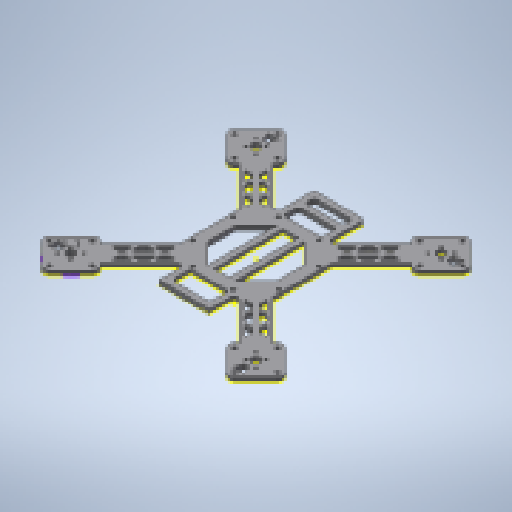
# Autodesk Inventor part: 顶板
Saved by Autodesk Inventor 2025.2 (Build 292293000, 293)
## iProperties
Created: 2025-10-21
Part Number: 顶板
Material: 常规
Document SubType Name: Modeling
Designer: BO‘S_SLAVE
Density: 1 g/cm^3
Appearance: 默认
Author: BO‘S_SLAVE
Autodesk Inventor part; units mm, degrees
ref_plane "YZ Plane" through (0, 0, 0) normal (1, 0, 0) x (0, 1, 0)
ref_plane "XZ Plane" through (0, 0, 0) normal (0, 1, 0) x (-1, 0, 0)
ref_plane "XY Plane" through (0, 0, 0) normal (0, 0, 1) x (1, 0, 0)
sketch "草图1" plane through (0, 0, 0) normal (0, 1, 0) x (-1, 0, 0)
  line L0 (27.5, 27.5) -> (-27.5, 27.5)
  line L1 (-27.5, 27.5) -> (-27.5, -27.5)
  line L2 (-27.5, -27.5) -> (27.5, -27.5)
  line L3 (27.5, -27.5) -> (27.5, 27.5)
  line L4 (77.7817, -77.7817) -> (-77.7817, 77.7817)
  line L5 (77.7817, 77.7817) -> (-77.7817, -77.7817)
  line L6 (0, 27.5) -> (0, -27.5)
  line L7 (27.5, 0) -> (-27.5, 0)
  line L8 (38.8909, 16.1091) -> (38.8909, -16.1091)
  line L9 (38.8909, -16.1091) -> (16.1091, -38.8909)
  line L10 (16.1091, -38.8909) -> (-16.1091, -38.8909)
  line L11 (-16.1091, -38.8909) -> (-38.8909, -16.1091)
  line L12 (-38.8909, -16.1091) -> (-38.8909, 16.1091)
  line L13 (-38.8909, 16.1091) -> (-16.1091, 38.8909)
  line L14 (-16.1091, 38.8909) -> (16.1091, 38.8909)
  line L15 (16.1091, 38.8909) -> (38.8909, 16.1091)
  line L16 (16.1091, -38.8909) -> (-16.1091, -38.8909)
  line L17 (-16.1091, 38.8909) -> (16.1091, 38.8909)
  line L18 (16.1091, 38.8909) -> (16.1091, 55)
  line L19 (-16.1091, 55) -> (-16.1091, 38.8909)
  line L20 (-70.7107, 84.8528) -> (-20.4289, 34.5711)
  line L21 (-34.5711, 20.4289) -> (-84.8528, 70.7107)
  line L22 (-84.8528, 70.7107) -> (-77.7817, 77.7817)
  line L23 (-77.7817, 77.7817) -> (-70.7107, 84.8528)
  line L24 (-53.033, 77.7817) -> (-77.7817, 53.033)
  line L25 (-77.7817, 53.033) -> (-102.5305, 77.7817)
  line L26 (-77.7817, 102.5305) -> (-53.033, 77.7817)
  line L27 (-53.033, 77.7817) -> (-102.5305, 77.7817) construction
  line L28 (-77.7817, 53.033) -> (-77.7817, 102.5305) construction
  line L29 (-11.3909, 27.5) -> (11.3909, 27.5)
  line L30 (11.3909, 27.5) -> (27.5, 11.3909)
  line L31 (27.5, 11.3909) -> (27.5, -11.3909)
  line L32 (27.5, -11.3909) -> (11.3909, -27.5)
  line L33 (11.3909, -27.5) -> (-11.3909, -27.5)
  line L34 (-11.3909, -27.5) -> (-27.5, -11.3909)
  line L35 (-27.5, -11.3909) -> (-27.5, 11.3909)
  line L36 (-27.5, 11.3909) -> (-11.3909, 27.5)
  line L37 (21.1091, 60) -> (21.1091, 33.8909)
  line L38 (-21.1091, 33.8909) -> (-21.1091, 60)
  circle A0 centre (-17, 36) radius 1.65
  line L39 (-38.8909, 0) -> (-27.5, 0)
  line L40 (0, 38.8909) -> (0, 27.5)
  line L41 (16.1091, 55) -> (-16.1091, 55)
  line L42 (21.1091, 60) -> (-21.1091, 60)
  circle A1 centre (-77.7817, 77.7817) radius 3.5
  circle A2 centre (-72.1249, 72.1249) radius 1.15
  circle A3 centre (-83.4386, 83.4386) radius 1.15
  circle A4 centre (-82.0244, 73.5391) radius 1.15
  circle A5 centre (-73.5391, 82.0244) radius 1.15
  circle A6 centre (-77.7817, 95.7817) radius 1.65
  circle A7 centre (-77.7817, 59.7817) radius 1.65
  circle A8 centre (-59.7817, 77.7817) radius 1.65
  circle A9 centre (-95.7817, 77.7817) radius 1.65
  line L43 (-77.7817, 102.5305) -> (-102.5305, 77.7817)
  line L44 (-77.7817, 102.5305) -> (-77.7817, 77.7817)
  line L45 (-77.7817, 77.7817) -> (-77.7817, 59.7817)
  line L46 (-73.5391, 82.0244) -> (-82.0244, 73.5391)
  line L47 (-72.1249, 72.1249) -> (-83.4386, 83.4386)
  line L48 (-20.4289, -34.5711) -> (-70.7107, -84.8528)
  line L49 (-84.8528, -70.7107) -> (-34.5711, -20.4289)
  line L50 (-77.7817, -53.033) -> (-53.033, -77.7817)
  line L51 (-102.5305, -77.7817) -> (-77.7817, -53.033)
  line L52 (-102.5305, -77.7817) -> (-77.7817, -102.5305)
  line L53 (-53.033, -77.7817) -> (-77.7817, -102.5305)
  line L54 (-82.0244, -73.5391) -> (-73.5391, -82.0244)
  circle A10 centre (-77.7817, -77.7817) radius 3.5
  circle A11 centre (-83.4386, -83.4386) radius 1.15
  circle A12 centre (-82.0244, -73.5391) radius 1.15
  circle A13 centre (-77.7817, -59.7817) radius 1.65
  circle A14 centre (-72.1249, -72.1249) radius 1.15
  circle A15 centre (-73.5391, -82.0244) radius 1.15
  circle A16 centre (-59.7817, -77.7817) radius 1.65
  circle A17 centre (-95.7817, -77.7817) radius 1.65
  circle A18 centre (-77.7817, -95.7817) radius 1.65
  line L55 (34.5711, -20.4289) -> (84.8528, -70.7107)
  line L56 (70.7107, -84.8528) -> (20.4289, -34.5711)
  line L57 (53.033, -77.7817) -> (77.7817, -53.033)
  line L58 (77.7817, -102.5305) -> (53.033, -77.7817)
  line L59 (77.7817, -102.5305) -> (102.5305, -77.7817)
  line L60 (77.7817, -53.033) -> (102.5305, -77.7817)
  line L61 (73.5391, -82.0244) -> (82.0244, -73.5391)
  circle A19 centre (77.7817, -77.7817) radius 3.5
  circle A20 centre (83.4386, -83.4386) radius 1.15
  circle A21 centre (73.5391, -82.0244) radius 1.15
  circle A22 centre (59.7817, -77.7817) radius 1.65
  circle A23 centre (72.1249, -72.1249) radius 1.15
  circle A24 centre (82.0244, -73.5391) radius 1.15
  circle A25 centre (77.7817, -59.7817) radius 1.65
  circle A26 centre (77.7817, -95.7817) radius 1.65
  circle A27 centre (95.7817, -77.7817) radius 1.65
  line L62 (20.4289, 34.5711) -> (70.7107, 84.8528)
  line L63 (84.8528, 70.7107) -> (34.5711, 20.4289)
  line L64 (77.7817, 53.033) -> (53.033, 77.7817)
  line L65 (102.5305, 77.7817) -> (77.7817, 53.033)
  line L66 (102.5305, 77.7817) -> (77.7817, 102.5305)
  line L67 (53.033, 77.7817) -> (77.7817, 102.5305)
  line L68 (82.0244, 73.5391) -> (73.5391, 82.0244)
  circle A28 centre (77.7817, 77.7817) radius 3.5
  circle A29 centre (83.4386, 83.4386) radius 1.15
  circle A30 centre (82.0244, 73.5391) radius 1.15
  circle A31 centre (77.7817, 59.7817) radius 1.65
  circle A32 centre (72.1249, 72.1249) radius 1.15
  circle A33 centre (73.5391, 82.0244) radius 1.15
  circle A34 centre (59.7817, 77.7817) radius 1.65
  circle A35 centre (95.7817, 77.7817) radius 1.65
  circle A36 centre (77.7817, 95.7817) radius 1.65
  circle A37 centre (-36, 17) radius 1.65
  circle A38 centre (-17, -36) radius 1.65
  circle A39 centre (-36, -17) radius 1.65
  circle A40 centre (17, 36) radius 1.65
  circle A41 centre (36, 17) radius 1.65
  circle A42 centre (36, -17) radius 1.65
  circle A43 centre (17, -36) radius 1.65
  line L69 (-19.4454, -19.4454) -> (-19.4454, 19.4454)
  line L70 (19.4454, -19.4454) -> (19.4454, 19.4454)
  line L71 (-16.1091, -38.8909) -> (-16.1091, -65)
  line L72 (-16.1091, -65) -> (16.1091, -65)
  line L73 (16.1091, -65) -> (16.1091, -38.8909)
  line L74 (-21.1091, -33.8909) -> (-21.1091, -70)
  line L75 (-21.1091, -70) -> (21.1091, -70)
  line L76 (21.1091, -70) -> (21.1091, -33.8909)
  line L77 (-16.1091, -56.9454) -> (16.1091, -56.9454)
  line L78 (-16.1091, -51.9454) -> (16.1091, -51.9454)
  line L79 (-11.5, 27.5) -> (-11.5, -27.5)
  line L80 (11.5, -27.5) -> (11.5, 27.5)
  line L81 (-6.5, -27.5) -> (-6.5, 27.5)
  line L82 (6.5, -27.5) -> (6.5, 27.5)
  line L83 (-63.9932, 66.8216) -> (-26.0858, 28.9142)
  line L84 (-66.8216, 63.9932) -> (-28.9142, 26.0858)
  line L85 (-58.3363, 72.4784) -> (-58.3363, 61.1647)
  line L86 (-56.3363, 70.4784) -> (-56.3363, 59.1647)
  line L87 (-42.1942, 56.3363) -> (-53.5079, 56.3363)
  line L88 (-40.1942, 54.3363) -> (-51.5079, 54.3363)
  line L89 (-40.1942, 54.3363) -> (-40.1942, 43.0226)
  line L90 (-38.1942, 52.2039) -> (-38.1942, 41.0226)
  line L91 (-35.3657, 38.1942) -> (-24.052, 38.1942)
  line L92 (-72.4784, 58.3363) -> (-61.1647, 58.3363)
  line L93 (-70.4784, 56.3363) -> (-59.1647, 56.3363)
  line L94 (-56.3363, 42.1942) -> (-56.3363, 53.5079)
  line L95 (-54.3363, 40.1942) -> (-54.3363, 51.5079)
  line L96 (-52.2039, 38.1942) -> (-41.0226, 38.1942)
  line L97 (-54.3363, 40.1942) -> (-43.0226, 40.1942)
  line L98 (-38.1942, 35.3657) -> (-38.1942, 24.052)
  line L99 (-70.3571, 60.4576) -> (-32.4497, 22.5503)
  line L100 (-60.4576, 70.3571) -> (-22.5503, 32.4497)
  line L101 (-38.1942, -35.3657) -> (-38.1942, -24.052)
  line L102 (-35.3657, -38.1942) -> (-24.052, -38.1942)
  line L103 (-38.1942, -52.2039) -> (-38.1942, -41.0226)
  line L104 (-40.1942, -54.3363) -> (-40.1942, -43.0226)
  line L105 (-52.2039, -38.1942) -> (-41.0226, -38.1942)
  line L106 (-54.3363, -40.1942) -> (-43.0226, -40.1942)
  line L107 (-60.4576, -70.3571) -> (-22.5503, -32.4497)
  line L108 (-42.1942, -56.3363) -> (-53.5079, -56.3363)
  line L109 (-40.1942, -54.3363) -> (-51.5079, -54.3363)
  line L110 (-56.3363, -70.4784) -> (-56.3363, -59.1647)
  line L111 (-58.3363, -72.4784) -> (-58.3363, -61.1647)
  line L112 (-63.9932, -66.8216) -> (-26.0858, -28.9142)
  line L113 (-66.8216, -63.9932) -> (-28.9142, -26.0858)
  line L114 (-70.4784, -56.3363) -> (-59.1647, -56.3363)
  line L115 (-72.4784, -58.3363) -> (-61.1647, -58.3363)
  line L116 (-70.3571, -60.4576) -> (-32.4497, -22.5503)
  line L117 (-56.3363, -42.1942) -> (-56.3363, -53.5079)
  line L118 (-54.3363, -40.1942) -> (-54.3363, -51.5079)
  line L119 (35.3657, -38.1942) -> (24.052, -38.1942)
  line L120 (38.1942, -35.3657) -> (38.1942, -24.052)
  line L121 (52.2039, -38.1942) -> (41.0226, -38.1942)
  line L122 (54.3363, -40.1942) -> (43.0226, -40.1942)
  line L123 (38.1942, -52.2039) -> (38.1942, -41.0226)
  line L124 (40.1942, -54.3363) -> (40.1942, -43.0226)
  line L125 (70.3571, -60.4576) -> (32.4497, -22.5503)
  line L126 (56.3363, -42.1942) -> (56.3363, -53.5079)
  line L127 (54.3363, -40.1942) -> (54.3363, -51.5079)
  line L128 (70.4784, -56.3363) -> (59.1647, -56.3363)
  line L129 (72.4784, -58.3363) -> (61.1647, -58.3363)
  line L130 (66.8216, -63.9932) -> (28.9142, -26.0858)
  line L131 (63.9932, -66.8216) -> (26.0858, -28.9142)
  line L132 (56.3363, -70.4784) -> (56.3363, -59.1647)
  line L133 (58.3363, -72.4784) -> (58.3363, -61.1647)
  line L134 (60.4576, -70.3571) -> (22.5503, -32.4497)
  line L135 (42.1942, -56.3363) -> (53.5079, -56.3363)
  line L136 (40.1942, -54.3363) -> (51.5079, -54.3363)
  line L137 (38.1942, 35.3657) -> (38.1942, 24.052)
  line L138 (35.3657, 38.1942) -> (24.052, 38.1942)
  line L139 (38.1942, 52.2039) -> (38.1942, 41.0226)
  line L140 (40.1942, 54.3363) -> (40.1942, 43.0226)
  line L141 (52.2039, 38.1942) -> (41.0226, 38.1942)
  line L142 (54.3363, 40.1942) -> (43.0226, 40.1942)
  line L143 (60.4576, 70.3571) -> (22.5503, 32.4497)
  line L144 (42.1942, 56.3363) -> (53.5079, 56.3363)
  line L145 (40.1942, 54.3363) -> (51.5079, 54.3363)
  line L146 (56.3363, 70.4784) -> (56.3363, 59.1647)
  line L147 (58.3363, 72.4784) -> (58.3363, 61.1647)
  line L148 (63.9932, 66.8216) -> (26.0858, 28.9142)
  line L149 (66.8216, 63.9932) -> (28.9142, 26.0858)
  line L150 (70.4784, 56.3363) -> (59.1647, 56.3363)
  line L151 (72.4784, 58.3363) -> (61.1647, 58.3363)
  line L152 (70.3571, 60.4576) -> (32.4497, 22.5503)
  line L153 (56.3363, 42.1942) -> (56.3363, 53.5079)
  line L154 (54.3363, 40.1942) -> (54.3363, 51.5079)
  line L155 (11.967, -28.8909) -> (-11.967, -28.8909)
  line L156 (-11.967, -28.8909) -> (-28.8909, -11.967)
  line L157 (-28.8909, -11.967) -> (-28.8909, 11.967)
  line L158 (-28.8909, 11.967) -> (-11.967, 28.8909)
  line L159 (-11.967, 28.8909) -> (11.967, 28.8909)
  line L160 (11.967, 28.8909) -> (28.8909, 11.967)
  line L161 (28.8909, 11.967) -> (28.8909, -11.967)
  line L162 (28.8909, -11.967) -> (11.967, -28.8909)
  line L163 (19.4454, -19.4454) -> (19.4454, -21.4124)
  line L164 (19.4454, 19.4454) -> (19.4454, 21.4124)
  line L165 (11.5, -27.5) -> (11.5, -28.8909)
  line L166 (6.5, -27.5) -> (6.5, -28.8909)
  line L167 (0, -27.5) -> (0, -28.8909)
  line L168 (19.4454, 19.4454) -> (19.4454, 21.4124)
  line L169 (11.5, 27.5) -> (11.5, 28.8909)
  line L170 (6.5, 27.5) -> (6.5, 28.8909)
  line L171 (0, 27.5) -> (0, 28.8909)
  line L172 (-19.4454, -19.4454) -> (-19.4454, -21.4124)
  line L173 (-19.4454, 19.4454) -> (-19.4454, 21.4124)
  line L174 (-11.5, -27.5) -> (-11.5, -28.8909)
  line L175 (-6.5, -27.5) -> (-6.5, -28.8909)
  line L176 (-11.5, 27.5) -> (-11.5, 28.8909)
  line L177 (-6.5, 27.5) -> (-6.5, 28.8909)
  line L178 (38.8909, -16.1091) -> (38.8909, -24.7487)
  line L179 (38.8909, 16.1091) -> (38.8909, 24.7487)
  line L180 (-38.8909, 16.1091) -> (-38.8909, 24.7487)
  line L181 (-38.8909, -24.7487) -> (-38.8909, -16.1091)
  line L182 (-83.7817, 77.7817) -> (-77.7817, 77.7817)
  line L183 (83.4484, 79.7817) -> (92.6247, 82.2405)
  line L184 (83.4484, 75.7817) -> (92.6247, 73.323)
  line L185 (83.4484, 75.7817) -> (83.4484, 79.7817)
  line L186 (77.7817, 77.7817) -> (77.7817, 102.5305)
  line L187 (84.9484, 75.3798) -> (84.9484, 80.1837)
  line L188 (83.4484, 77.7817) -> (77.7817, 77.7817)
  line L189 (92.6247, 73.323) -> (92.6247, 82.2405)
  line L190 (-75.7817, 83.4484) -> (-73.323, 92.6247)
  line L191 (-73.323, 92.6247) -> (-82.2405, 92.6247)
  line L192 (-79.7817, 83.4484) -> (-82.2405, 92.6247)
  line L193 (-75.3798, 84.9484) -> (-80.1837, 84.9484)
  line L194 (-75.7817, 83.4484) -> (-79.7817, 83.4484)
  line L195 (-83.4484, -75.7817) -> (-92.6247, -73.323)
  line L196 (-92.6247, -73.323) -> (-92.6247, -82.2405)
  line L197 (-83.4484, -79.7817) -> (-92.6247, -82.2405)
  line L198 (-84.9484, -75.3798) -> (-84.9484, -80.1837)
  line L199 (-83.4484, -75.7817) -> (-83.4484, -79.7817)
  line L200 (75.7817, -83.4484) -> (73.323, -92.6247)
  line L201 (73.323, -92.6247) -> (82.2405, -92.6247)
  line L202 (79.7817, -83.4484) -> (82.2405, -92.6247)
  line L203 (75.3798, -84.9484) -> (80.1837, -84.9484)
  line L204 (75.7817, -83.4484) -> (79.7817, -83.4484)
  arc A44 (88.4163, 74.97) -> (88.4163, 80.5935) centre (77.7817, 77.7817) ccw construction
  point P0 (0, 0)
  point P1 (0, 0)
  point P2 (0, 0)
  point P3 (0, 0)
  point P4 (-77.7817, 77.7817)
  point P5 (0, 0)
  point P6 (-72.4784, 58.3363)
  point P7 (22.5736, 37.4264)
  point P8 (-21.1091, 33.8909)
  point P9 (-59.7505, 71.0642)
  point P10 (16.1091, 38.8909)
  point P11 (-11.3909, 27.5)
  point P12 (11.3909, 27.5)
  point P13 (-77.7817, 77.7817)
  point P14 (-72.7259, 82.8376)
  point P15 (-74.0198, 81.0909)
  point P16 (-81.0909, 74.0198)
  point P17 (-82.8376, 72.7259)
  point P18 (-75.3069, 80.2566)
  point P19 (-80.2566, 75.3069)
  point P20 (-77.7817, -77.7817)
  point P21 (77.7817, -77.7817)
  point P22 (77.7817, 77.7817)
  point P23 (20.4289, -34.5711)
  point P24 (58.3363, -72.4784)
  point P25 (72.4784, -58.3363)
  point P26 (34.5711, -20.4289)
  point P27 (34.5711, 20.4289)
  point P28 (72.4784, 58.3363)
  point P29 (58.3363, 72.4784)
  point P30 (20.4289, 34.5711)
  point P31 (-58.3363, -72.4784)
  point P32 (-20.4289, -34.5711)
  point P33 (-34.5711, -20.4289)
  point P34 (-72.4784, -58.3363)
  point P35 (16.1091, 38.8909)
  point P36 (15.8157, -30)
  point P37 (18.1843, -30)
  point P38 (18.1843, 30)
  point P39 (15.8157, 30)
  point P40 (-18.1843, -30)
  point P41 (-15.8157, -30)
  point P42 (9.3198, -22.5)
  point P43 (9.3198, -22.5)
  point P44 (27.5, 11.3909)
  point P45 (27.5, -11.3909)
  point P46 (-9.3198, -22.5)
  point P47 (11.5, 27.5)
  point P48 (-11.5, 27.5)
  point P49 (-11.5, -30)
  point P50 (11.5, -30)
  point P51 (11.5, 27.3909)
  point P52 (11.5, -27.3909)
  point P53 (-11.5, 27.3909)
  point P54 (-11.5, -27.3909)
  point P55 (-6.5, -27.5)
  point P56 (-6.5, 27.5)
  point P57 (6.5, 27.5)
  point P58 (6.5, -27.5)
  point P59 (-74.3523, 81.2112)
  point P60 (-81.2112, 74.3523)
  point P61 (-29.7089, 38.1942)
  point P62 (-38.1942, 35.3657)
  point P63 (-38.1942, 28.2947)
  point P64 (-48.0937, 38.1942)
  point P65 (-41.0226, 38.1942)
  point P66 (-54.3363, 51.5079)
  point P67 (-43.0226, 40.1942)
  point P68 (-50.0937, 40.1942)
  point P69 (-54.3363, 44.4368)
  point P70 (-59.1647, 56.3363)
  point P71 (-56.3363, 53.5079)
  point P72 (-56.3363, 46.4368)
  point P73 (-66.2358, 56.3363)
  point P74 (-56.3363, 66.2358)
  point P75 (-46.4368, 56.3363)
  point P76 (-28.2947, 38.1942)
  point P77 (-38.1942, 48.0937)
  point P78 (-44.4368, 54.3363)
  point P79 (-40.1942, 50.0937)
  point P80 (-61.1647, 58.3363)
  point P81 (-68.2358, 58.3363)
  point P82 (-58.3363, 68.2358)
  point P83 (-21.1091, -35.2513)
  point P84 (21.1091, -35.2513)
  point P85 (-21.1091, 35.2513)
  point P86 (-38.1942, -29.7089)
  point P87 (29.7089, -38.1942)
  point P88 (38.1942, 29.7089)
  point P89 (0, 0)
  point P90 (0, -38.8909)
  point P91 (0, -28.8909)
  point P92 (40.1942, 50.0937)
  point P93 (44.4368, 54.3363)
  point P94 (38.1942, 28.2947)
  point P95 (48.0937, 38.1942)
  point P96 (68.2358, 58.3363)
  point P97 (54.3363, 44.4368)
  point P98 (50.0937, 40.1942)
  point P99 (66.2358, 56.3363)
  point P100 (56.3363, 46.4368)
  point P101 (58.3363, 68.2358)
  point P102 (46.4368, 56.3363)
  point P103 (56.3363, 66.2358)
  point P104 (28.2947, 38.1942)
  point P105 (38.1942, 48.0937)
  point P106 (6.5, 28.8909)
  point P107 (-6.5, -28.8909)
  point P108 (-6.5, 28.8909)
  point P109 (-32.4497, -22.5503)
  point P110 (-38.1942, -28.2947)
  point P111 (-11.5, 28.8909)
  point P112 (-11.5, -28.8909)
  point P113 (11.5, 28.8909)
  point P114 (-68.2358, -58.3363)
  point P115 (-58.3363, -68.2358)
  point P116 (58.3363, -68.2358)
  point P117 (68.2358, -58.3363)
  point P118 (-28.2947, -38.1942)
  point P119 (-38.1942, -48.0937)
  point P120 (-46.4368, -56.3363)
  point P121 (-56.3363, -66.2358)
  point P122 (-48.0937, -38.1942)
  point P123 (-50.0937, -40.1942)
  point P124 (-54.3363, -44.4368)
  point P125 (-66.2358, -56.3363)
  point P126 (-56.3363, -46.4368)
  point P127 (-40.1942, -50.0937)
  point P128 (-44.4368, -54.3363)
  point P129 (38.1942, -28.2947)
  point P130 (48.0937, -38.1942)
  point P131 (56.3363, -46.4368)
  point P132 (66.2358, -56.3363)
  point P133 (50.0937, -40.1942)
  point P134 (54.3363, -44.4368)
  point P135 (28.2947, -38.1942)
  point P136 (38.1942, -48.0937)
  point P137 (40.1942, -50.0937)
  point P138 (44.4368, -54.3363)
  point P139 (56.3363, -66.2358)
  point P140 (46.4368, -56.3363)
  point P141 (21.1091, 35.2513)
  point P142 (-22.5503, -32.4497)
  point P143 (-58.3363, -72.4784)
  point P144 (22.5503, -32.4497)
  point P145 (26.0858, -28.9142)
  point P146 (58.3363, -72.4784)
  point P147 (28.9142, -26.0858)
  point P148 (32.4497, -22.5503)
  point P149 (72.4784, -58.3363)
  point P150 (58.3363, -72.4784)
  point P151 (-72.4784, -58.3363)
  point P152 (-72.4784, -58.3363)
  point P153 (72.4784, -58.3363)
  point P154 (-58.3363, -72.4784)
  point P155 (11.5, 24.3579)
  point P156 (11.5, -24.3579)
  point P157 (-11.5, -24.3579)
  point P158 (-11.5, 24.3579)
  point P159 (-77.7817, 61.4317)
  point P160 (-78.0517, 63.9095)
  point P161 (-77.7817, 63.6396)
  point P162 (11.5, 27.5)
  point P163 (-37.601, 17.399)
  point P164 (-36.399, 18.601)
  point P165 (36.399, 18.601)
  point P166 (37.601, 17.399)
  point P167 (37.601, -17.399)
  point P168 (36.399, -18.601)
  point P169 (17.399, 37.601)
  point P170 (18.601, 36.399)
  point P171 (-18.601, 36.399)
  point P172 (-17.399, 37.601)
  point P173 (-37.601, -17.399)
  point P174 (-36.399, -18.601)
  point P175 (-77.7817, 83.4484)
  point P176 (-83.4484, -77.7817)
  point P177 (77.7817, -83.4484)
  dimension "d6" = 220
  dimension "d7" = 55
  dimension "d8" = 45
  dimension "d9" = 45
  dimension "d12" = 10
  dimension "d13" = 10
  dimension "d21" = 5
  dimension "d22" = 5
  dimension "d30" = 3.3
  dimension "d31" = 36
  dimension "d33" = 17
  dimension "d46" = 5
  dimension "d50" = 7
  dimension "d51" = 2.3
  dimension "d52" = 2.3
  dimension "d55" = 2.3
  dimension "d56" = 2.3
  dimension "d58" = 6
  dimension "d67" = 3.3
  dimension "d68" = 3.3
  dimension "d71" = 35
  dimension "d72" = 35
  dimension "d73" = 18
  dimension "d74" = 36
  dimension "d77" = 6
  dimension "d78" = 16
  dimension "d79" = 8
  dimension "d82" = 360
  dimension "d88" = 3.3
  dimension "d90" = 17
  dimension "d91" = 8.5
  dimension "d95" = 55
  dimension "d96" = 5
  dimension "d98" = 5
  dimension "d99" = 5
  dimension "d100" = 65
  dimension "d101" = 5
  dimension "d110" = 23
  dimension "d112" = 11.5
  dimension "d113" = 5
  dimension "d116" = 2
  dimension "d117" = 2
  dimension "d118" = 45
  dimension "d119" = 2
  dimension "d120" = 4
  dimension "d121" = 2
  dimension "d122" = 45
  dimension "d124" = 2
  dimension "d127" = 45
  dimension "d128" = 45
  dimension "d129" = 4
  dimension "d139" = 3
  dimension "d140" = 3
  dimension "d153" = 360
  dimension "d155" = 10
  dimension "d164" = 105
  dimension "d165" = 105
  dimension "d166" = 5.6667
  dimension "d167" = 1.5
  dimension "d168" = 9.5
  dimension "d169" = 4
  dimension "d172" = 360
  constraints: 402 end point, 51 point on line, 45 centre point, 32 symmetric about line, 27 midpoint, 19 perpendicular, 18 parallel, 8 collinear, 7 coincident, 5 horizontal, 5 vertical, 3 equal length, 2 point on circle, 499 other
  measures "d6" distance of L5.start L5.end
  measures "d7" distance of L2.start L3.start
  measures "d8" angle of L6 L5
  measures "d9" angle of L6 L4
  measures "d12" distance of L22.end L23.end
  measures "d13" distance of L22.start L22.end
  measures "d21" distance between parallel lines of L19 L38
  measures "d22" distance between parallel lines of L18 L37
  measures "d30" diameter of A0
  measures "d31" distance from line of L39 A0.centre
  measures "d33" distance from line of L6 A0.centre
  measures "d46" distance between parallel lines of L41 L42
  measures "d50" diameter of A1
  measures "d51" diameter of A2
  measures "d52" diameter of A3
  measures "d55" diameter of A5
  measures "d56" diameter of A4
  measures "d58" distance of A1.centre L46.start
  measures "d67" diameter of A7
  measures "d68" diameter of A6
  measures "d71" distance of L26.start L27.end
  measures "d72" distance of L26.start L24.start
  measures "d73" distance of point (-77.782, 77.782) A6.centre
  measures "d74" distance of A6.centre L45.end
  measures "d77" distance of L46.end point (-77.782, 77.782)
  measures "d78" distance of L47.end L47.start
  measures "d79" distance of L182.end L47.start
  measures "d88" diameter of A37
  measures "d90" distance from line of L7 A37.centre
  measures "d91" distance from line of L35 A37.centre
  measures "d95" distance between parallel lines of L41 L7
  measures "d96" distance between parallel lines of L71 L74
  measures "d98" distance between parallel lines of L73 L76
  measures "d99" distance between parallel lines of L72 L75
  measures "d100" distance between parallel lines of L7 L72
  measures "d101" distance between parallel lines of L78 L77
  measures "d110" distance between parallel lines of L80 L79
  measures "d112" distance between parallel lines of L6 L80
  measures "d113" distance between parallel lines of L79 L81
  measures "d116" distance from line of L4 point (-63.993, 66.822)
  measures "d117" distance between parallel lines of L4 L84
  measures "d119" distance between parallel lines of L85 L86
  measures "d120" distance of L86.end L87.end
  measures "d121" distance between parallel lines of L88 L87
  measures "d124" distance between parallel lines of L89 L90
  measures "d129" distance of L90.end L91.start
  measures "d139" distance between parallel lines of L20 L100
  measures "d140" distance between parallel lines of L99 L21
  measures "d155" distance of point (0, -38.891) point (0, -28.891)
  measures "d164" angle of L185 L184
  measures "d165" angle of L185 L183
  measures "d166" distance between parallel lines of L185 L186
  measures "d167" distance between parallel lines of L187 L185
  measures "d168" distance of L184.start L184.end
  measures "d169" distance of L184.start L183.start
extrude "拉伸1" add sketch "草图1" along normal blind 4 contours L80 L30 L0 | L0 L170 L159 L169 | L30 L80 L5 L82 L0 | L160 L159 L40 L14 L15 A40 L0 | L0 L5 L160 | L15 A41 L8 L9 A42 L3 L162 L161 L160 | L15 L148 L64 L5 | L3 L160 L5 | L5 L64 L149 L15 | L80 L7 L82 L5 | L64 L67 L186 A36 A28 L5 A32 | L185 L183 L187 L184 | L5 A32 A28 L186 A36 L66 L65 L64 | L15 L143 L138 L148 | L149 L137 L152 L15 | L80 L4 L82 L7 | L159 L158 L0 L13 A0 L14 L40 | L81 L4 L79 L36 L0 | L0 L176 L159 L177 | L64 L152 L151 L149 | L148 L147 L143 L64 | L15 L37 L62 L138 L143 | L152 L137 L63 L15 | L80 L32 L2 L82 L4 | L36 L79 L0 | L81 L7 L79 L4 | L81 L2 L34 L79 L5 | L5 L79 L7 L81 | L64 L151 L152 | L151 L152 L150 L149 | L143 L147 L64 | L148 L146 L143 L147 | L15 L62 L37 | L138 L62 L140 L143 | L139 L143 L140 L148 | L63 L179 L15 A41 | L152 L142 L63 L137 | L149 L142 L152 L141 | L162 L3 L4 | L4 L2 L162 | L80 L2 L32 | L13 A0 L20 L38 L42 L37 L62 L15 A40 L18 L41 L19 | L2 L165 L155 L166 | L175 L155 L174 L2 | L155 L162 L2 L9 A43 L10 L11 A38 L156 | L63 L150 L152 L151 | L147 L143 L146 L62 | L9 L130 L57 L4 | L4 L57 L131 L9 | L158 L4 L0 | L34 L2 L79 | L63 L153 L152 L150 | L153 L152 L154 L149 | L146 L143 L144 L62 | L148 L145 L143 L144 | L145 L143 L140 | L62 L144 L143 L145 | L152 L154 L142 | L57 L60 L59 L58 | L9 L125 L120 L130 | L131 L119 L134 L9 | L4 L158 L1 | L13 L84 L24 L4 | L1 L158 L157 L39 L12 L13 A37 | L4 L24 L83 L13 | L156 L2 L5 | L5 L1 L156 | L63 L154 L152 L153 | L57 L134 L133 L131 | L130 L129 L125 L57 | L9 L55 L120 L125 | L134 L119 L56 L76 L9 | L13 L38 L20 | L24 L21 L45 A1 L4 A2 | L4 A2 A1 L23 A5 L20 L24 | L13 L99 L98 L84 | L83 L91 L100 L13 | L11 A39 L12 L39 L157 L156 L1 | L11 L112 L50 L5 | L5 L50 L113 L11 | L38 L13 L100 L91 L20 | L178 L55 L9 A42 | L57 L133 L134 | L133 L134 L132 L131 | L125 L129 L57 | L130 L128 L125 L129 | L120 L55 L122 L125 | L121 L125 L122 L130 | L76 L56 L9 | L134 L124 L56 L119 | L131 L124 L134 L123 | L24 L100 L85 L83 | L84 L92 L99 L24 | L13 L21 L98 L99 | L50 L53 L52 L51 | L11 L107 L102 L112 | L113 L101 L116 L11 | L91 L100 L89 L20 | L56 L132 L134 L133 | L129 L125 L128 L55 | L56 L76 L75 L74 L48 L11 A38 L71 L72 L73 L9 A43 | L24 L85 L100 | L85 L100 L86 L83 | L99 L92 L24 | L84 L93 L99 L92 | L13 A37 L180 L21 | L98 L21 L97 L99 | L96 L99 L97 L84 | L83 L89 L100 L90 | L50 L116 L115 L113 | L112 L111 L107 L50 | L11 L74 L48 L102 L107 | L116 L101 L49 L11 | L11 A39 L49 L181 | L88 L100 L87 L20 | L89 L100 L88 | L127 L125 L122 | L55 L126 L125 L127 | L56 L135 L134 L132 | L135 L134 L136 L131 | L128 L125 L126 L55 | L130 L127 L125 L126 | L136 L134 L135 L56 | L124 L134 L136 | L20 L23 A5 A1 L44 L194 L190 L191 A6 L26 L24 | L20 L86 L100 L85 | L92 L99 L93 L21 | L24 L25 L43 L44 A6 L191 L192 L194 A1 L22 A4 L21 | L50 L115 L116 | L115 L116 L114 L113 | L107 L111 L50 | L112 L110 L107 L111 | L11 L48 L74 | L102 L48 L104 L107 | L103 L107 L104 L112 | L116 L106 L49 L101 | L113 L106 L116 L105 | L11 A39 | L87 L100 L86 L20 | L88 L83 L87 L100 | L45 L21 L22 A4 A1 | L93 L99 L94 L21 | L84 L95 L99 L94 | L97 L95 L99 | L49 L114 L116 L115 | L111 L107 L110 L48 | L118 L116 L117 L49 | L106 L116 L118 | L21 L94 L99 L95 | L49 L117 L116 L114 | L117 L116 L118 L113 | L110 L107 L108 L48 | L112 L109 L107 L108 | L109 L107 L104 | L48 L108 L107 L109 | L73 L77 L71 L78 | L194 L192 L193 L44 | L44 L193 L190 L194 | L199 L197 L198 L195 | L204 L202 L203 L200 picked at (-37.1593, -17.9112)
fillet "圆角2" radius 5 16 edges at (102.5305, 2, -77.7817) (77.7817, 2, -53.033) (53.033, 2, -77.7817) (77.7817, 2, -102.5305) (-77.7817, 2, -102.5305) (-102.5305, 2, -77.7817) (-77.7817, 2, -53.033) (-77.7817, 2, 102.5305) (-102.5305, 2, 77.7817) (-77.7817, 2, 53.033) (-53.033, 2, 77.7817) (77.7817, 2, 102.5305) (53.033, 2, 77.7817) (77.7817, 2, 53.033) (102.5305, 2, 77.7817) (-53.033, 2, -77.7817)
fillet "圆角4" radius 2 2 edges at (21.1091, 2, -70) (-21.1091, 2, -70)
fillet "圆角6" radius 1 23 edges at (-38.1942, 2, 28.2947) (-28.2947, 2, 38.1942) (-53.5079, 2, 56.3363) (-40.1942, 2, 43.0226) (-35.3657, 2, 38.1942) (-50.0937, 2, 40.1942) (-56.3363, 2, 46.4368) (-56.3363, 2, 66.2358) (-66.2358, 2, 56.3363) (-51.5079, 2, 54.3363) (-38.1942, 2, 41.0226) (-54.3363, 2, 44.4368) (-48.0937, 2, 38.1942) (-38.1942, 2, 48.0937) (-41.0226, 2, 38.1942) (-54.3363, 2, 51.5079) (-44.4368, 2, 54.3363) (-38.1942, 2, 35.3657) (-43.0226, 2, 40.1942) (-40.1942, 2, 50.0937) (-56.3363, 2, 53.5079) (-46.4368, 2, 56.3363) (-56.3363, 2, 59.1647)
fillet "圆角7" radius 1 24 edges at (-28.2947, 2, -38.1942) (-38.1942, 2, -28.2947) (-50.0937, 2, -40.1942) (-40.1942, 2, -50.0937) (-46.4368, 2, -56.3363) (-56.3363, 2, -53.5079) (-53.5079, 2, -56.3363) (-40.1942, 2, -43.0226) (-35.3657, 2, -38.1942) (-56.3363, 2, -46.4368) (-56.3363, 2, -59.1647) (-66.2358, 2, -56.3363) (-54.3363, 2, -44.4368) (-48.0937, 2, -38.1942) (-41.0226, 2, -38.1942) (-59.1647, 2, -56.3363) (-54.3363, 2, -51.5079) (-43.0226, 2, -40.1942) (-38.1942, 2, -35.3657) (-56.3363, 2, -66.2358) (-44.4368, 2, -54.3363) (-51.5079, 2, -54.3363) (-38.1942, 2, -41.0226) (-38.1942, 2, -48.0937)
fillet "圆角8" radius 1 24 edges at (38.1942, 2, -35.3657) (41.0226, 2, -38.1942) (38.1942, 2, -28.2947) (35.3657, 2, -38.1942) (50.0937, 2, -40.1942) (40.1942, 2, -43.0226) (56.3363, 2, -46.4368) (53.5079, 2, -56.3363) (56.3363, 2, -53.5079) (43.0226, 2, -40.1942) (28.2947, 2, -38.1942) (38.1942, 2, -48.0937) (38.1942, 2, -41.0226) (48.0937, 2, -38.1942) (54.3363, 2, -44.4368) (66.2358, 2, -56.3363) (59.1647, 2, -56.3363) (54.3363, 2, -51.5079) (51.5079, 2, -54.3363) (40.1942, 2, -50.0937) (44.4368, 2, -54.3363) (56.3363, 2, -59.1647) (46.4368, 2, -56.3363) (56.3363, 2, -66.2358)
fillet "圆角9" radius 1 23 edges at (56.3363, 2, 66.2358) (44.4368, 2, 54.3363) (38.1942, 2, 48.0937) (38.1942, 2, 41.0226) (51.5079, 2, 54.3363) (56.3363, 2, 59.1647) (28.2947, 2, 38.1942) (46.4368, 2, 56.3363) (40.1942, 2, 50.0937) (53.5079, 2, 56.3363) (40.1942, 2, 43.0226) (35.3657, 2, 38.1942) (59.1647, 2, 56.3363) (56.3363, 2, 53.5079) (43.0226, 2, 40.1942) (38.1942, 2, 35.3657) (38.1942, 2, 28.2947) (48.0937, 2, 38.1942) (54.3363, 2, 44.4368) (66.2358, 2, 56.3363) (56.3363, 2, 46.4368) (54.3363, 2, 51.5079) (41.0226, 2, 38.1942)
fillet "圆角10" radius 3 12 edges at (-16.1091, 2, -38.8909) (16.1091, 2, -38.8909) (16.1091, 2, -51.9454) (-16.1091, 2, -51.9454) (-16.1091, 2, -65) (16.1091, 2, -65) (16.1091, 2, -56.9454) (-16.1091, 2, -56.9454) (16.1091, 2, 38.8909) (-16.1091, 2, 38.8909) (-16.1091, 2, 55) (16.1091, 2, 55)
fillet "圆角11" radius 3 4 edges at (-21.1091, 2, -35.2513) (21.1091, 2, -35.2513) (21.1091, 2, 35.2513) (-21.1091, 2, 35.2513)
sketch "草图2" plane through (0, 0, 0) normal (0, -1, 0) x (1, 0, 0)
  line L0 (-40.7297, -37.9013) -> (-38.4871, -35.6586) projected
  line L1 (-39.9013, -30.0018) -> (-46.3866, -36.4871) projected
  circle A0 centre (-59.7817, -77.7817) radius 1.65 projected
  circle A1 centre (-77.7817, -59.7817) radius 1.65 projected
  circle A2 centre (-95.7817, -77.7817) radius 1.65 projected
  circle A3 centre (-77.7817, -95.7817) radius 1.65 projected
  circle A4 centre (-83.4386, -83.4386) radius 1.15 projected
  circle A5 centre (-72.1249, -72.1249) radius 1.15 projected
  circle A6 centre (-77.7817, -77.7817) radius 3.5 projected
  circle A7 centre (-82.0244, -73.5391) radius 1.15 projected
  circle A8 centre (-73.5391, -82.0244) radius 1.15 projected
  line L2 (46.3866, -36.4871) -> (39.9013, -30.0018) projected
  line L3 (38.4871, -35.6586) -> (40.7297, -37.9013) projected
  line L4 (11.5, -28.8909) -> (11.967, -28.8909) projected
  line L5 (11.967, 28.8909) -> (11.5, 28.8909) projected
  line L6 (-53.8008, -56.6292) -> (-56.0434, -58.8718) projected
  line L7 (-54.6292, -64.5287) -> (-48.1439, -58.0434) projected
  circle A9 centre (-36, 17) radius 1.65 projected
  circle A10 centre (-36, -17) radius 1.65 projected
  circle A11 centre (-17, 36) radius 1.65 projected
  line L8 (56.0434, -58.8718) -> (53.8008, -56.6292) projected
  line L9 (48.1439, -58.0434) -> (54.6292, -64.5287) projected
  circle A12 centre (17, 36) radius 1.65 projected
  line L10 (58.0434, 48.1439) -> (64.5287, 54.6292) projected
  line L11 (58.8718, 56.0434) -> (56.6292, 53.8008) projected
  circle A13 centre (36, 17) radius 1.65 projected
  line L12 (72.4784, 58.3363) -> (38.8909, 24.7487) projected
  circle A14 centre (72.1249, 72.1249) radius 1.15 projected
  circle A15 centre (77.7817, 77.7817) radius 3.5 projected
  line L13 (6.5, -28.8909) -> (6.5, 28.8909) projected
  line L14 (-6.5, 28.8909) -> (-6.5, -28.8909) projected
  circle A16 centre (83.4386, -83.4386) radius 1.15 projected
  circle A17 centre (77.7817, -59.7817) radius 1.65 projected
  circle A18 centre (59.7817, -77.7817) radius 1.65 projected
  circle A19 centre (95.7817, -77.7817) radius 1.65 projected
  circle A20 centre (77.7817, -95.7817) radius 1.65 projected
  circle A21 centre (73.5391, -82.0244) radius 1.15 projected
  circle A22 centre (82.0244, -73.5391) radius 1.15 projected
  circle A23 centre (72.1249, -72.1249) radius 1.15 projected
  circle A24 centre (77.7817, -77.7817) radius 3.5 projected
  arc A25 (-21.1091, -68) -> (-19.1091, -70) centre (-19.1091, -68) ccw projected
  line L15 (19.1091, -70) -> (-19.1091, -70) projected
  arc A26 (19.1091, -70) -> (21.1091, -68) centre (19.1091, -68) ccw projected
  line L16 (21.1091, -42.4939) -> (21.1091, -68) projected
  arc A27 (26.2304, -40.3726) -> (21.1091, -42.4939) centre (24.1091, -42.4939) ccw projected
  line L17 (58.3363, -72.4784) -> (26.2304, -40.3726) projected
  line L18 (56.5685, -74.2462) -> (58.3363, -72.4784) projected
  arc A28 (56.5685, -74.2462) -> (56.5685, -81.3173) centre (60.1041, -77.7817) ccw projected
  line L19 (74.2462, -98.9949) -> (56.5685, -81.3173) projected
  arc A29 (74.2462, -98.9949) -> (81.3173, -98.9949) centre (77.7817, -95.4594) ccw projected
  line L20 (98.9949, -81.3173) -> (81.3173, -98.9949) projected
  arc A30 (98.9949, -81.3173) -> (98.9949, -74.2462) centre (95.4594, -77.7817) ccw projected
  line L21 (81.3173, -56.5685) -> (98.9949, -74.2462) projected
  arc A31 (81.3173, -56.5685) -> (74.2462, -56.5685) centre (77.7817, -60.1041) ccw projected
  line L22 (72.4784, -58.3363) -> (74.2462, -56.5685) projected
  line L23 (38.8909, -24.7487) -> (72.4784, -58.3363) projected
  line L24 (38.8909, 24.7487) -> (38.8909, -24.7487) projected
  line L25 (74.2462, 56.5685) -> (72.4784, 58.3363) projected
  arc A32 (74.2462, 56.5685) -> (81.3173, 56.5685) centre (77.7817, 60.1041) ccw projected
  line L26 (98.9949, 74.2462) -> (81.3173, 56.5685) projected
  arc A33 (98.9949, 74.2462) -> (98.9949, 81.3173) centre (95.4594, 77.7817) ccw projected
  line L27 (81.3173, 98.9949) -> (98.9949, 81.3173) projected
  arc A34 (81.3173, 98.9949) -> (74.2462, 98.9949) centre (77.7817, 95.4594) ccw projected
  line L28 (56.5685, 81.3173) -> (74.2462, 98.9949) projected
  arc A35 (56.5685, 81.3173) -> (56.5685, 74.2462) centre (60.1041, 77.7817) ccw projected
  line L29 (58.3363, 72.4784) -> (56.5685, 74.2462) projected
  line L30 (26.2304, 40.3726) -> (58.3363, 72.4784) projected
  arc A36 (21.1091, 42.4939) -> (26.2304, 40.3726) centre (24.1091, 42.4939) ccw projected
  line L31 (21.1091, 60) -> (21.1091, 42.4939) projected
  line L32 (-21.1091, 60) -> (21.1091, 60) projected
  line L33 (-21.1091, 42.4939) -> (-21.1091, 60) projected
  arc A37 (-26.2304, 40.3726) -> (-21.1091, 42.4939) centre (-24.1091, 42.4939) ccw projected
  line L34 (-58.3363, 72.4784) -> (-26.2304, 40.3726) projected
  line L35 (-56.5685, 74.2462) -> (-58.3363, 72.4784) projected
  arc A38 (-56.5685, 74.2462) -> (-56.5685, 81.3173) centre (-60.1041, 77.7817) ccw projected
  line L36 (-74.2462, 98.9949) -> (-56.5685, 81.3173) projected
  arc A39 (-74.2462, 98.9949) -> (-81.3173, 98.9949) centre (-77.7817, 95.4594) ccw projected
  line L37 (-98.9949, 81.3173) -> (-81.3173, 98.9949) projected
  arc A40 (-98.9949, 81.3173) -> (-98.9949, 74.2462) centre (-95.4594, 77.7817) ccw projected
  line L38 (-81.3173, 56.5685) -> (-98.9949, 74.2462) projected
  arc A41 (-81.3173, 56.5685) -> (-74.2462, 56.5685) centre (-77.7817, 60.1041) ccw projected
  line L39 (-72.4784, 58.3363) -> (-74.2462, 56.5685) projected
  line L40 (-38.8909, 24.7487) -> (-72.4784, 58.3363) projected
  line L41 (-38.8909, -24.7487) -> (-38.8909, 24.7487) projected
  line L42 (-72.4784, -58.3363) -> (-38.8909, -24.7487) projected
  line L43 (-74.2462, -56.5685) -> (-72.4784, -58.3363) projected
  arc A42 (-74.2462, -56.5685) -> (-81.3173, -56.5685) centre (-77.7817, -60.1041) ccw projected
  line L44 (-98.9949, -74.2462) -> (-81.3173, -56.5685) projected
  arc A43 (-98.9949, -74.2462) -> (-98.9949, -81.3173) centre (-95.4594, -77.7817) ccw projected
  line L45 (-81.3173, -98.9949) -> (-98.9949, -81.3173) projected
  arc A44 (-81.3173, -98.9949) -> (-74.2462, -98.9949) centre (-77.7817, -95.4594) ccw projected
  line L46 (-56.5685, -81.3173) -> (-74.2462, -98.9949) projected
  arc A45 (-56.5685, -81.3173) -> (-56.5685, -74.2462) centre (-60.1041, -77.7817) ccw projected
  line L47 (-58.3363, -72.4784) -> (-56.5685, -74.2462) projected
  line L48 (-26.2304, -40.3726) -> (-58.3363, -72.4784) projected
  arc A46 (-21.1091, -42.4939) -> (-26.2304, -40.3726) centre (-24.1091, -42.4939) ccw projected
  line L49 (-21.1091, -68) -> (-21.1091, -42.4939) projected
  line L50 (-16.1091, 52) -> (-16.1091, 38.8909) projected
  arc A47 (-13.1091, 55) -> (-16.1091, 52) centre (-13.1091, 52) ccw projected
  line L51 (13.1091, 55) -> (-13.1091, 55) projected
  arc A48 (16.1091, 52) -> (13.1091, 55) centre (13.1091, 52) ccw projected
  line L52 (16.1091, 41.8909) -> (16.1091, 52) projected
  arc A49 (13.1091, 38.8909) -> (16.1091, 41.8909) centre (13.1091, 41.8909) ccw projected
  line L53 (-16.1091, 38.8909) -> (13.1091, 38.8909) projected
  circle A50 centre (-88.7817, 66.7817) radius 1.65
  line L54 (-77.7817, 77.7817) -> (-88.7817, 66.7817)
  circle A51 centre (-77.7817, 95.7817) radius 1.65 projected
  circle A52 centre (-77.7817, 77.7817) radius 18
  arc A53 (48.851, -56.3363) -> (48.1439, -58.0434) centre (48.851, -57.3363) ccw projected
  line L55 (53.0937, -56.3363) -> (48.851, -56.3363) projected
  arc A54 (53.8008, -56.6292) -> (53.0937, -56.3363) centre (53.0937, -57.3363) ccw projected
  arc A55 (56.3363, -59.579) -> (56.0434, -58.8718) centre (55.3363, -59.579) ccw projected
  line L56 (56.3363, -63.8216) -> (56.3363, -59.579) projected
  arc A56 (54.6292, -64.5287) -> (56.3363, -63.8216) centre (55.3363, -63.8216) ccw projected
  line L57 (37.9013, -40.7297) -> (35.6586, -38.4871) projected
  line L58 (30.0018, -39.9013) -> (36.4871, -46.3866) projected
  arc A57 (-56.0434, -58.8718) -> (-56.3363, -59.579) centre (-55.3363, -59.579) ccw projected
  arc A58 (-53.0937, -56.3363) -> (-53.8008, -56.6292) centre (-53.0937, -57.3363) ccw projected
  line L59 (-48.851, -56.3363) -> (-53.0937, -56.3363) projected
  arc A59 (-48.1439, -58.0434) -> (-48.851, -56.3363) centre (-48.851, -57.3363) ccw projected
  arc A60 (-56.3363, -63.8216) -> (-54.6292, -64.5287) centre (-55.3363, -63.8216) ccw projected
  line L60 (-56.3363, -59.579) -> (-56.3363, -63.8216) projected
  line L61 (-44.1439, -54.0434) -> (-40.4871, -50.3866) projected
  line L62 (-41.9013, -44.7297) -> (-49.8008, -52.6292) projected
  arc A61 (59.579, 56.3363) -> (58.8718, 56.0434) centre (59.579, 55.3363) ccw projected
  line L63 (63.8216, 56.3363) -> (59.579, 56.3363) projected
  arc A62 (64.5287, 54.6292) -> (63.8216, 56.3363) centre (63.8216, 55.3363) ccw projected
  arc A63 (56.3363, 48.851) -> (58.0434, 48.1439) centre (57.3363, 48.851) ccw projected
  line L64 (56.3363, 53.0937) -> (56.3363, 48.851) projected
  arc A64 (56.6292, 53.8008) -> (56.3363, 53.0937) centre (57.3363, 53.0937) ccw projected
  line L65 (52.6292, 49.8008) -> (44.7297, 41.9013) projected
  line L66 (50.0937, 40.1942) -> (54.0434, 44.1439) projected
  line L67 (6.5, 28.8909) -> (-6.5, 28.8909) projected
  line L68 (-6.5, -28.8909) -> (6.5, -28.8909) projected
  line L69 (11.5, 28.8909) -> (11.5, -28.8909) projected
  line L70 (28.8909, 11.967) -> (11.967, 28.8909) projected
  line L71 (28.8909, -11.967) -> (28.8909, 11.967) projected
  line L72 (11.967, -28.8909) -> (28.8909, -11.967) projected
  arc A65 (30.7089, -38.1942) -> (30.0018, -39.9013) centre (30.7089, -39.1942) ccw projected
  line L73 (34.9515, -38.1942) -> (30.7089, -38.1942) projected
  arc A66 (35.6586, -38.4871) -> (34.9515, -38.1942) centre (34.9515, -39.1942) ccw projected
  arc A67 (38.1942, -41.4368) -> (37.9013, -40.7297) centre (37.1942, -41.4368) ccw projected
  line L74 (38.1942, -45.6795) -> (38.1942, -41.4368) projected
  arc A68 (36.4871, -46.3866) -> (38.1942, -45.6795) centre (37.1942, -45.6795) ccw projected
  arc A69 (-49.6795, -40.1942) -> (-50.3866, -40.4871) centre (-49.6795, -41.1942) ccw projected
  line L75 (-45.4368, -40.1942) -> (-49.6795, -40.1942) projected
  arc A70 (-44.7297, -41.9013) -> (-45.4368, -40.1942) centre (-45.4368, -41.1942) ccw projected
  line L76 (-52.6292, -49.8008) -> (-44.7297, -41.9013) projected
  arc A71 (-54.3363, -49.0937) -> (-52.6292, -49.8008) centre (-53.3363, -49.0937) ccw projected
  line L77 (-54.3363, -44.851) -> (-54.3363, -49.0937) projected
  arc A72 (-54.0434, -44.1439) -> (-54.3363, -44.851) centre (-53.3363, -44.851) ccw projected
  line L78 (-50.3866, -40.4871) -> (-54.0434, -44.1439) projected
  arc A73 (-40.4871, -50.3866) -> (-40.1942, -49.6795) centre (-41.1942, -49.6795) ccw projected
  arc A74 (-44.851, -54.3363) -> (-44.1439, -54.0434) centre (-44.851, -53.3363) ccw projected
  line L79 (-49.0937, -54.3363) -> (-44.851, -54.3363) projected
  arc A75 (-49.8008, -52.6292) -> (-49.0937, -54.3363) centre (-49.0937, -53.3363) ccw projected
  arc A76 (-40.1942, -45.4368) -> (-41.9013, -44.7297) centre (-41.1942, -45.4368) ccw projected
  line L80 (-40.1942, -49.6795) -> (-40.1942, -45.4368) projected
  arc A77 (-30.0018, -39.9013) -> (-30.7089, -38.1942) centre (-30.7089, -39.1942) ccw projected
  line L81 (-36.4871, -46.3866) -> (-30.0018, -39.9013) projected
  arc A78 (-38.1942, -45.6795) -> (-36.4871, -46.3866) centre (-37.1942, -45.6795) ccw projected
  line L82 (-38.1942, -41.4368) -> (-38.1942, -45.6795) projected
  arc A79 (-37.9013, -40.7297) -> (-38.1942, -41.4368) centre (-37.1942, -41.4368) ccw projected
  line L83 (-35.6586, -38.4871) -> (-37.9013, -40.7297) projected
  arc A80 (-34.9515, -38.1942) -> (-35.6586, -38.4871) centre (-34.9515, -39.1942) ccw projected
  line L84 (-30.7089, -38.1942) -> (-34.9515, -38.1942) projected
  arc A81 (-56.3363, -48.851) -> (-58.0434, -48.1439) centre (-57.3363, -48.851) ccw projected
  line L85 (-56.3363, -53.0937) -> (-56.3363, -48.851) projected
  arc A82 (-56.6292, -53.8008) -> (-56.3363, -53.0937) centre (-57.3363, -53.0937) ccw projected
  line L86 (-58.8718, -56.0434) -> (-56.6292, -53.8008) projected
  arc A83 (-59.579, -56.3363) -> (-58.8718, -56.0434) centre (-59.579, -55.3363) ccw projected
  line L87 (-63.8216, -56.3363) -> (-59.579, -56.3363) projected
  arc A84 (-64.5287, -54.6292) -> (-63.8216, -56.3363) centre (-63.8216, -55.3363) ccw projected
  line L88 (-58.0434, -48.1439) -> (-64.5287, -54.6292) projected
  arc A85 (-38.1942, -30.7089) -> (-39.9013, -30.0018) centre (-39.1942, -30.7089) ccw projected
  line L89 (-38.1942, -34.9515) -> (-38.1942, -30.7089) projected
  arc A86 (-38.4871, -35.6586) -> (-38.1942, -34.9515) centre (-39.1942, -34.9515) ccw projected
  arc A87 (-41.4368, -38.1942) -> (-40.7297, -37.9013) centre (-41.4368, -37.1942) ccw projected
  line L90 (-45.6795, -38.1942) -> (-41.4368, -38.1942) projected
  arc A88 (-46.3866, -36.4871) -> (-45.6795, -38.1942) centre (-45.6795, -37.1942) ccw projected
  arc A89 (58.8718, -56.0434) -> (59.579, -56.3363) centre (59.579, -55.3363) ccw projected
  line L91 (56.6292, -53.8008) -> (58.8718, -56.0434) projected
  arc A90 (56.3363, -53.0937) -> (56.6292, -53.8008) centre (57.3363, -53.0937) ccw projected
  line L92 (56.3363, -48.851) -> (56.3363, -53.0937) projected
  arc A91 (58.0434, -48.1439) -> (56.3363, -48.851) centre (57.3363, -48.851) ccw projected
  line L93 (64.5287, -54.6292) -> (58.0434, -48.1439) projected
  arc A92 (63.8216, -56.3363) -> (64.5287, -54.6292) centre (63.8216, -55.3363) ccw projected
  line L94 (59.579, -56.3363) -> (63.8216, -56.3363) projected
  arc A93 (50.3866, -40.4871) -> (49.6795, -40.1942) centre (49.6795, -41.1942) ccw projected
  line L95 (54.0434, -44.1439) -> (50.3866, -40.4871) projected
  arc A94 (54.3363, -44.851) -> (54.0434, -44.1439) centre (53.3363, -44.851) ccw projected
  line L96 (54.3363, -49.0937) -> (54.3363, -44.851) projected
  arc A95 (52.6292, -49.8008) -> (54.3363, -49.0937) centre (53.3363, -49.0937) ccw projected
  line L97 (44.7297, -41.9013) -> (52.6292, -49.8008) projected
  arc A96 (45.4368, -40.1942) -> (44.7297, -41.9013) centre (45.4368, -41.1942) ccw projected
  line L98 (49.6795, -40.1942) -> (45.4368, -40.1942) projected
  arc A97 (39.9013, -30.0018) -> (38.1942, -30.7089) centre (39.1942, -30.7089) ccw projected
  arc A98 (45.6795, -38.1942) -> (46.3866, -36.4871) centre (45.6795, -37.1942) ccw projected
  line L99 (41.4368, -38.1942) -> (45.6795, -38.1942) projected
  arc A99 (40.7297, -37.9013) -> (41.4368, -38.1942) centre (41.4368, -37.1942) ccw projected
  arc A100 (38.1942, -34.9515) -> (38.4871, -35.6586) centre (39.1942, -34.9515) ccw projected
  line L100 (38.1942, -30.7089) -> (38.1942, -34.9515) projected
  arc A101 (40.1942, -49.6795) -> (40.4871, -50.3866) centre (41.1942, -49.6795) ccw projected
  line L101 (40.1942, -45.4368) -> (40.1942, -49.6795) projected
  arc A102 (41.9013, -44.7297) -> (40.1942, -45.4368) centre (41.1942, -45.4368) ccw projected
  line L102 (49.8008, -52.6292) -> (41.9013, -44.7297) projected
  arc A103 (49.0937, -54.3363) -> (49.8008, -52.6292) centre (49.0937, -53.3363) ccw projected
  line L103 (44.851, -54.3363) -> (49.0937, -54.3363) projected
  arc A104 (44.1439, -54.0434) -> (44.851, -54.3363) centre (44.851, -53.3363) ccw projected
  line L104 (40.4871, -50.3866) -> (44.1439, -54.0434) projected
  arc A105 (41.4368, 38.1942) -> (40.7297, 37.9013) centre (41.4368, 37.1942) ccw projected
  line L105 (45.6795, 38.1942) -> (41.4368, 38.1942) projected
  arc A106 (46.3866, 36.4871) -> (45.6795, 38.1942) centre (45.6795, 37.1942) ccw projected
  line L106 (39.9013, 30.0018) -> (46.3866, 36.4871) projected
  arc A107 (38.1942, 30.7089) -> (39.9013, 30.0018) centre (39.1942, 30.7089) ccw projected
  line L107 (38.1942, 34.9515) -> (38.1942, 30.7089) projected
  arc A108 (38.4871, 35.6586) -> (38.1942, 34.9515) centre (39.1942, 34.9515) ccw projected
  line L108 (40.7297, 37.9013) -> (38.4871, 35.6586) projected
  arc A109 (54.3363, 49.0937) -> (52.6292, 49.8008) centre (53.3363, 49.0937) ccw projected
  line L109 (54.3363, 44.851) -> (54.3363, 49.0937) projected
  arc A110 (54.0434, 44.1439) -> (54.3363, 44.851) centre (53.3363, 44.851) ccw projected
  line L110 (45.4368, 40.1942) -> (50.0937, 40.1942) projected
  arc A111 (44.7297, 41.9013) -> (45.4368, 40.1942) centre (45.4368, 41.1942) ccw projected
  point P0 (0, 0)
  dimension "d157" = 3.3
  constraints: 2 coincident, 2 end point, 1 centre point, 1 parallel, 1 vertical alignment, 2 other
  measures "d157" diameter of A50
